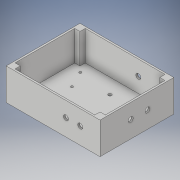
# Autodesk Inventor part: 546-1590BBS-ADF41020
Saved by Autodesk Inventor 2018 (Build 220112000, 112)
## iProperties
Created: 2018-04-27
Part Number: 546-1590BBS-ADF41020
Material: Generic
Document SubType Name: Modeling
Designer: bbramman
Density: 1 g/cm^3
Appearance: Default
Author: bbramman
Autodesk Inventor part; units mm, degrees
ref_plane "YZ Plane" through (0, 0, 0) normal (1, 0, 0) x (0, 1, 0)
ref_plane "XZ Plane" through (0, 0, 0) normal (0, 1, 0) x (-1, 0, 0)
ref_plane "XY Plane" through (0, 0, 0) normal (0, 0, 1) x (1, 0, 0)
sketch "Sketch1" plane through (0, 0, 0) normal (0, 1, 0) x (-1, 0, 0)
  line L0 (-59.7535, -47.0027) -> (59.7535, -47.0027)
  line L1 (59.7535, -47.0027) -> (59.7535, 47.0027)
  line L2 (59.7535, 47.0027) -> (-59.7535, 47.0027)
  line L3 (-59.7535, 47.0027) -> (-59.7535, -47.0027)
  line L4 (-59.7535, -47.0027) -> (59.7535, 47.0027) construction
  line L5 (59.7535, -47.0027) -> (-59.7535, 47.0027) construction
  point P0 (0, 0)
  dimension "d0" = 119.507
  dimension "d1" = 94.0054
  constraints: 12 end point, 2 midpoint, 2 parallel, 1 horizontal, 1 perpendicular
  measures "d0" distance of L2.end L1.end
  measures "d1" distance of L1.end L0.end
extrude "Extrusion1" add sketch "Sketch1" along normal mid plane 2.2606
sketch "Sketch2" plane through (0, 1.1303, 0) normal (0, 1, 0) x (1, 0, 0)
  line L0 (-59.7535, 47.0027) -> (-59.7535, -47.0027) projected
  line L1 (59.7535, -47.0027) -> (59.7535, 47.0027) projected
  line L2 (-59.7535, -47.0027) -> (59.7535, -47.0027)
  line L3 (59.7535, -47.0027) -> (59.7535, 47.0027)
  line L4 (59.7535, 47.0027) -> (-59.7535, 47.0027)
  line L5 (-59.7535, 47.0027) -> (-59.7535, -47.0027)
  line L6 (57.4929, -44.7421) -> (-57.4929, 44.7421) construction
  line L7 (-57.4929, -44.7421) -> (57.4929, 44.7421) construction
  line L8 (-59.7535, -47.0027) -> (59.7535, -47.0027) projected
  line L9 (-59.7535, -47.0027) -> (-50.7619, -47.0027)
  line L10 (-59.7535, -38.0111) -> (-59.7535, -47.0027)
  line L11 (-59.7535, 47.0027) -> (-50.7619, 47.0027)
  line L12 (-59.7535, 38.0111) -> (-59.7535, 47.0027)
  line L13 (59.7535, 47.0027) -> (-59.7535, 47.0027) projected
  line L14 (59.7535, 47.0027) -> (50.7619, 47.0027)
  line L15 (59.7535, 38.0111) -> (59.7535, 47.0027)
  line L16 (59.7535, -47.0027) -> (50.7619, -47.0027)
  line L17 (59.7535, -38.0111) -> (59.7535, -47.0027)
  line L18 (-50.7619, -44.7421) -> (-50.7619, -38.0111)
  line L19 (-50.7619, -38.0111) -> (-57.4929, -38.0111)
  line L20 (-57.4929, 38.0111) -> (-50.7619, 38.0111)
  line L21 (-50.7619, 38.0111) -> (-50.7619, 44.7421)
  line L22 (50.7619, 38.0111) -> (57.4929, 38.0111)
  line L23 (50.7619, 44.7421) -> (50.7619, 38.0111)
  line L24 (57.4929, -38.0111) -> (50.7619, -38.0111)
  line L25 (50.7619, -38.0111) -> (50.7619, -44.7421)
  line L26 (-50.7619, -44.7421) -> (50.7619, -44.7421)
  line L27 (57.4929, -38.0111) -> (57.4929, 38.0111)
  line L28 (50.7619, 44.7421) -> (-50.7619, 44.7421)
  line L29 (-57.4929, 38.0111) -> (-57.4929, -38.0111)
  point P0 (0, 0)
  dimension "d4" = 114.9858
  dimension "d5" = 89.4842
  dimension "d6" = 8.9916
  dimension "d7" = 8.9916
  dimension "d10" = 8.9916
  dimension "d11" = 8.9916
  constraints: 52 end point, 7 horizontal, 3 perpendicular, 2 midpoint, 2 parallel
  measures "d4" distance of L6.end L7.end
  measures "d5" distance of L7.start L6.end
  measures "d6" distance of L10.start L18.end
  measures "d7" distance of L18.end L9.end
  measures "d10" distance of L15.start L22.start
  measures "d11" distance of L22.start L14.end
extrude "Extrusion2" add sketch "Sketch2" along normal blind 38.1
sketch "Sketch3" plane through (0, 1.1303, 0) normal (0, 1, 0) x (1, 0, 0)
  circle A0 centre (0, -25.4) radius 2.0828
  circle A1 centre (0, 25.4) radius 2.0828
  point P0 (0, 0)
  dimension "d18" = 4.1656
  dimension "d19" = 4.1656
  constraints: 2 centre point
  measures "d18" diameter of A0
  measures "d19" diameter of A1
extrude "Extrusion3" cut sketch "Sketch3" against normal through all
sketch "Sketch7" plane through (0, 1.1303, 0) normal (0, 1, 0) x (1, 0, 0)
  line L0 (44.9961, -32.4993) -> (-44.9961, 32.4993) construction
  line L1 (-44.9961, -32.4993) -> (44.9961, 32.4993) construction
  line L2 (-44.9961, -32.4993) -> (-38.6461, -32.4993) construction
  line L3 (44.9961, -32.4993) -> (64.0461, -32.4993) construction
  line L4 (32.9946, -9.9949) -> (-32.9946, 9.9949) construction
  line L5 (-32.9946, -9.9949) -> (32.9946, 9.9949) construction
  circle A0 centre (-32.9946, -9.9949) radius 1.4986
  circle A1 centre (-32.9946, 9.9949) radius 1.4986
  circle A2 centre (32.9946, -9.9949) radius 1.4986
  circle A3 centre (32.9946, 9.9949) radius 1.4986
  line L6 (-44.45, -32.1469) -> (44.45, -32.1469)
  line L7 (44.45, 32.1469) -> (-44.45, 32.1469)
  line L8 (-44.45, 32.1469) -> (-44.45, -32.1469)
  line L9 (-44.45, -32.1469) -> (44.45, 32.1469) construction
  line L10 (44.45, -32.1469) -> (-44.45, 32.1469) construction
  line L11 (-44.45, -32.1469) -> (-43.434, -32.1469)
  line L12 (-44.45, -31.1309) -> (-44.45, -32.1469)
  circle A4 centre (-43.434, -31.1309) radius 1.524
  line L13 (-44.45, 32.1469) -> (-43.434, 32.1469)
  line L14 (-44.45, 31.1309) -> (-44.45, 32.1469)
  circle A5 centre (-43.434, 31.1309) radius 1.524
  line L15 (44.45, 32.1469) -> (43.434, 32.1469)
  line L16 (44.45, 31.1309) -> (44.45, 32.1469)
  circle A6 centre (43.434, 31.1309) radius 1.524
  line L17 (44.45, -32.1469) -> (43.434, -32.1469)
  line L18 (43.434, -31.1309) -> (44.45, -31.1309)
  circle A7 centre (43.434, -31.1309) radius 1.524
  point P0 (0, 0)
  dimension "d47" = 89.9922
  dimension "d48" = 64.9986
  dimension "d62" = 65.9892
  dimension "d63" = 19.9898
  dimension "d64" = 2.9972
  dimension "d65" = 2.9972
  dimension "d66" = 2.9972
  dimension "d67" = 2.9972
  dimension "d120" = 88.9
  dimension "d121" = 64.2938
  dimension "d124" = 3.048
  dimension "d127" = 3.048
  dimension "d130" = 3.048
  dimension "d131" = 1.016
  dimension "d132" = 1.016
  dimension "d133" = 3.048
  constraints: 38 end point, 8 centre point, 7 horizontal, 6 midpoint, 5 coincident, 2 parallel
  measures "d47" distance of L0.end L1.end
  measures "d48" distance of L1.start L0.end
  measures "d62" distance of L4.end L5.end
  measures "d63" distance of L5.start L4.end
  measures "d64" diameter of A0
  measures "d65" diameter of A1
  measures "d66" diameter of A2
  measures "d67" diameter of A3
  measures "d120" distance of L7.end L7.start
  measures "d121" distance of L7.start L6.end
  measures "d124" diameter of A4
  measures "d127" diameter of A5
  measures "d130" diameter of A6
  measures "d131" distance of L18.start L18.end
  measures "d132" distance of L17.end L18.start
  measures "d133" diameter of A7
sketch "Sketch8" plane through (-50.7619, 1.1303, -44.7421) normal (0, 0, 1) x (1, 0, 0)
  line L0 (0, 0) -> (0, 38.1) projected
  circle A0 centre (67.6783, 19.05) radius 3.175
  point P0 (50.7619, -1.1303)
  dimension "d99" = 6.35
  constraints: 1 centre point
  measures "d99" diameter of A0
extrude "Extrusion7" cut sketch "Sketch8" against normal through all
sketch "Sketch10" plane through (57.4929, 1.1303, -38.0111) normal (-1, 0, 0) x (0, 0, 1)
  line L0 (0, 0) -> (0, 38.1) projected
  line L1 (0, 19.05) -> (5.5118, 19.05) construction
  circle A0 centre (24.5618, 19.05) radius 3.175
  circle A1 centre (45.993, 19.05) radius 3.175
  point P0 (38.0111, -1.1303)
  dimension "d118" = 6.35
  dimension "d119" = 6.35
  constraints: 2 centre point, 2 end point, 1 horizontal, 1 midpoint
  measures "d118" diameter of A0
  measures "d119" diameter of A1
extrude "Extrusion8" cut sketch "Sketch10" against normal through all
sketch "Sketch11" plane through (50.7619, 1.1303, 44.7421) normal (0, 0, -1) x (-1, 0, 0)
  line L0 (101.5238, 0) -> (101.5238, 38.1) projected
  line L1 (101.5238, 19.05) -> (95.758, 19.05)
  line L2 (0, 0) -> (0, 38.1) projected
  line L3 (0, 0) -> (0, 38.1) projected
  circle A0 centre (16.0846, 19.05) radius 3.175
  circle A1 centre (34.3408, 19.05) radius 3.175
  point P0 (50.7619, -1.1303)
  dimension "d80" = 5.7658
  dimension "d112" = 6.35
  dimension "d113" = 6.35
  constraints: 2 centre point, 2 end point, 1 horizontal, 1 midpoint
  measures "d80" distance of L1.start L1.end
  measures "d112" diameter of A0
  measures "d113" diameter of A1
extrude "Extrusion9" cut sketch "Sketch11" against normal through all
extrude "Extrusion10" cut sketch "Sketch7" against normal through all
body "Solid1"
